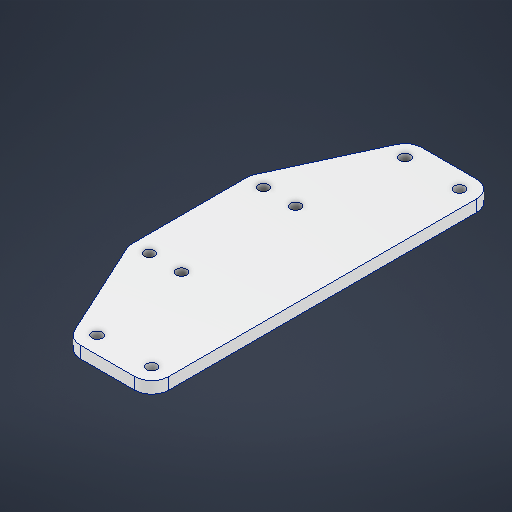
# Autodesk Inventor part: CNC-017-SpindleMountPlate2
Saved by Autodesk Inventor 2026.2 (Build 302298000, 298)
## iProperties
Created: 2026-06-22
Part Number: CNC-017-SpindleMountPlate2
Material: Aluminum 6061
Document SubType Name: Modeling
Designer: Kenji
Density: 2.7 g/cm^3
Appearance: Aluminum - Flat
Author: Kenji
Autodesk Inventor part; units mm, degrees
ref_plane "YZ Plane" through (0, 0, 0) normal (1, 0, 0) x (0, 1, 0)
ref_plane "XZ Plane" through (0, 0, 0) normal (0, 1, 0) x (-1, 0, 0)
ref_plane "XY Plane" through (0, 0, 0) normal (0, 0, 1) x (1, 0, 0)
sketch "Sketch1" plane through (0, 0, 0) normal (0, 1, 0) x (-1, 0, 0)
  circle A0 centre (0, 0) radius 2.1
  circle A1 centre (13, 0) radius 2.1
  circle A2 centre (13, 46) radius 2.1
  circle A3 centre (0, 46) radius 2.1
  circle A4 centre (-5, -39) radius 2.1
  circle A5 centre (-5, 85) radius 2.1
  circle A6 centre (-27, -39) radius 2.1
  circle A7 centre (-27, 85) radius 2.1
  circle A8 centre (13, 46) radius 6.8625 construction
  circle A9 centre (13, 0) radius 6.8625 construction
  circle A10 centre (-5, -39) radius 6.8625 construction
  circle A11 centre (-5, 85) radius 6.8625 construction
  circle A12 centre (-27, 85) radius 6.8625 construction
  circle A13 centre (-27, -39) radius 6.8625 construction
  line L0 (19.2309, -2.8758) -> (1.2309, -41.8758)
  line L1 (1.2309, 87.8758) -> (19.2309, 48.8758)
  line L2 (-5, 91.8625) -> (-27, 91.8625)
  line L3 (-5, -45.8625) -> (-27, -45.8625)
  line L4 (-33.8625, 85) -> (-33.8625, -39)
  line L5 (19.8625, 46) -> (19.8625, 0)
  arc A14 (19.2309, -2.8758) -> (19.8625, 0) centre (13, 0) ccw
  arc A15 (-5, -45.8625) -> (1.2309, -41.8758) centre (-5, -39) ccw
  arc A16 (-33.8625, -39) -> (-27, -45.8625) centre (-27, -39) ccw
  arc A17 (-27, 91.8625) -> (-33.8625, 85) centre (-27, 85) ccw
  arc A18 (1.2309, 87.8758) -> (-5, 91.8625) centre (-5, 85) ccw
  arc A19 (19.8625, 46) -> (19.2309, 48.8758) centre (13, 46) ccw
  dimension "d0" = 4.2
  dimension "d1" = 13
  dimension "d2" = 46
  dimension "d3" = 39
  dimension "d4" = 5
  dimension "d5" = 39
  dimension "d8" = 22
  dimension "d9" = 4.7625
  constraints: 24 point on circle, 20 centre point, 17 equal radius, 13 tangent, 12 end point, 6 coincident, 4 horizontal alignment, 4 vertical alignment, 2 vertical, 1 horizontal
  measures "d0" diameter of A0
  measures "d1" distance of point (0, 0) A1.centre
  measures "d2" distance of A1.centre A2.centre
  measures "d3" vertical distance of point (0, 0) A4.centre
  measures "d4" horizontal distance of A4.centre point (0, 0)
  measures "d5" vertical distance of A5.centre A3.centre
  measures "d8" distance of A6.centre A4.centre
  measures "d9" radial gap between concentric circles of A2 A8
extrude "Extrusion1" add sketch "Sketch1" along normal blind 4.7625
equation "\"d5\" = d3"
body "Solid1"
